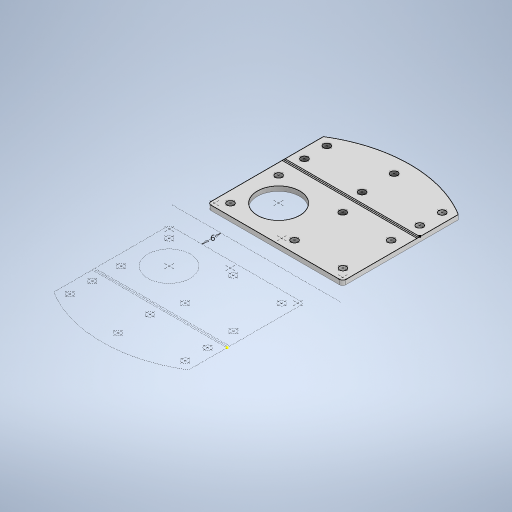
# Autodesk Inventor part: axis_2_bottom_L_frame(bottom)
Saved by Autodesk Inventor 2024.2 (Build 282272000, 272)
## iProperties
Created: 2024-01-11
Part Number: axis_2_bottom_L_frame(bottom)
Material: Generic
Document SubType Name: Modeling
Designer: chanh
Density: 1 g/cm^3
Appearance: Default
Author: chanh
Autodesk Inventor part; units mm, degrees
ref_plane "YZ Plane" through (0, 0, 0) normal (1, 0, 0) x (0, 1, 0)
ref_plane "XZ Plane" through (0, 0, 0) normal (0, 1, 0) x (-1, 0, 0)
ref_plane "XY Plane" through (0, 0, 0) normal (0, 0, 1) x (1, 0, 0)
sketch "Sketch1" plane through (0, 0, 0) normal (0, 1, 0) x (-1, 0, 0)
  line L0 (42.1, -0.4496) -> (0, -0.4496) construction
  circle A0 centre (31.1, -13.0193) radius 6.6 construction
  circle A1 centre (38.6, -20.5443) radius 1.05 construction
  circle A2 centre (38.6, -5.4943) radius 1.05 construction
  circle A3 centre (18.6, -5.4943) radius 1.05 construction
  circle A4 centre (18.6, -20.5443) radius 1.05 construction
  circle A5 centre (3.5, -20.5443) radius 1.05 construction
  circle A6 centre (3.5, -5.4943) radius 1.05 construction
  circle A7 centre (3.05, 10) radius 1.05 construction
  circle A8 centre (3.05, 3) radius 1.05 construction
  circle A9 centre (21.05, 3) radius 1.05 construction
  circle A10 centre (21.05, 13) radius 1.05 construction
  circle A11 centre (39.05, 10) radius 1.05 construction
  circle A12 centre (39.05, 3) radius 1.05 construction
  arc A13 (41.1, -24.0893) -> (42.1, -23.0893) centre (41.1, -23.0893) ccw construction
  line L1 (41.1, -24.0893) -> (1, -24.0893) construction
  arc A14 (0, -23.0893) -> (1, -24.0893) centre (1, -23.0893) ccw construction
  arc A15 (42.1, 11.9532) -> (0, 11.9532) centre (21.05, -22.06) ccw construction
  line L2 (0, -23.0893) -> (0, 11.9532) construction
  line L3 (42.1, 11.9532) -> (42.1, -23.0893) construction
  line L4 (42.1, -0.8993) -> (0, -0.8993) construction
  line L5 (0, 0) -> (42.1, 0) construction
  line L6 (47.4315, -30.0893) -> (-5.3631, -30.0893) construction
  line L7 (42.1, -59.7289) -> (0, -59.7289)
  circle A16 centre (31.1, -47.1593) radius 6.6
  circle A17 centre (38.6, -39.6343) radius 1.05
  circle A18 centre (38.6, -54.6843) radius 1.05
  circle A19 centre (18.6, -54.6843) radius 1.05
  circle A20 centre (18.6, -39.6343) radius 1.05
  circle A21 centre (3.5, -39.6343) radius 1.05
  circle A22 centre (3.5, -54.6843) radius 1.05
  circle A23 centre (3.05, -70.1786) radius 1.05
  circle A24 centre (3.05, -63.1786) radius 1.05
  circle A25 centre (21.05, -63.1786) radius 1.05
  circle A26 centre (21.05, -73.1786) radius 1.05
  circle A27 centre (39.05, -70.1786) radius 1.05
  circle A28 centre (39.05, -63.1786) radius 1.05
  arc A29 (42.1, -37.0893) -> (41.1, -36.0893) centre (41.1, -37.0893) ccw
  line L8 (41.1, -36.0893) -> (1, -36.0893)
  arc A30 (1, -36.0893) -> (0, -37.0893) centre (1, -37.0893) ccw
  arc A31 (0, -72.1318) -> (42.1, -72.1318) centre (21.05, -38.1186) ccw
  line L9 (0, -37.0893) -> (0, -72.1318)
  line L10 (42.1, -72.1318) -> (42.1, -37.0893)
  line L11 (42.1, -59.2793) -> (0, -59.2793)
  line L12 (0, -60.1786) -> (42.1, -60.1786)
  dimension "d0" = 6
  constraints: 32 centre point, 29 symmetric about line, 26 end point, 12 point on circle, 12 point on line, 5 horizontal, 2 vertical, 61 other
  measures "d0" distance between parallel lines of L6 L1
extrude "Extrusion1" add sketch "Sketch1" against normal blind 1.5
body "Solid1"
